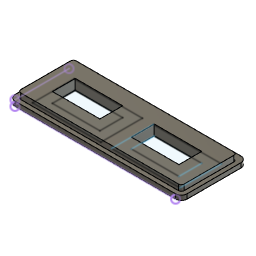
1593LBK_frontplate (Autodesk Fusion 360 design; units mm, degrees)
Autodesk Fusion 360 part; units mm, degrees
sketch "Skizze1" plane through (0, 0, 0) normal (0, 1, 0) x (1, 0, 0)
  arc A0 (0, 2) -> (2, 0) centre (2, 2) ccw
  arc A1 (2, 23) -> (0, 21) centre (2, 21) ccw
  line L0 (58.5, 23) -> (2, 23)
  line L1 (60.5, 2) -> (60.5, 21)
  arc A2 (58.5, 0) -> (60.5, 2) centre (58.5, 2) ccw
  line L2 (2, 0) -> (58.5, 0)
  line L3 (0, 21) -> (0, 2)
  arc A3 (60.5, 21) -> (58.5, 23) centre (58.5, 21) ccw
  point P0 (60.5, 0)
  point P1 (0, 23)
  dimension "d1" = 60.5
  dimension "d2" = 23
  dimension "d3" = 2
  dimension "d4" = 2
  dimension "d5" = 2
  dimension "d6" = 2
  constraint horizontal L2
  constraint vertical L1
  constraint horizontal L0
  constraint vertical L3
  constraint tangent L1 A3
  constraint tangent L0 A3
  constraint coincident P0 L2
  constraint coincident P0 L1
  constraint tangent A2 L2
  constraint tangent L1 A2
  constraint coincident origin L2
  constraint coincident origin L3
  constraint tangent A0 L2
  constraint tangent A0 L3
  constraint coincident P1 L0
  constraint coincident P1 L3
  constraint tangent A1 L0
  constraint tangent A1 L3
  measures "d1" distance of origin P0
  measures "d2" distance of origin P1
  measures "d3" radius of A3
  measures "d4" radius of A2
  measures "d5" radius of A0
  measures "d6" radius of A1
sketch "Skizze2" plane through (0, 0, 0) normal (0, 1, 0) x (1, 0, 0)
  line L0 (2.5, 1.5) -> (58, 1.5)
  line L1 (59, 2.5) -> (59, 20)
  line L2 (58, 21) -> (2.5, 21)
  line L3 (1.5, 20) -> (1.5, 2.5)
  line L4 (2, 0) -> (58.5, 0)
  line L5 (0, 21) -> (0, 2)
  arc A0 (2.5, 21) -> (1.5, 20) centre (2.5, 20) ccw
  arc A1 (1.5, 2.5) -> (2.5, 1.5) centre (2.5, 2.5) ccw
  arc A2 (59, 20) -> (58, 21) centre (58, 20) ccw
  arc A3 (58, 1.5) -> (59, 2.5) centre (58, 2.5) ccw
  point P0 (1.5, 1.5)
  point P1 (59, 1.5)
  point P2 (1.5, 21)
  dimension "d7" = 57.5
  dimension "d8" = 19.5
  dimension "d9" = 1.5
  dimension "d10" = 1.5
  dimension "d11" = 1
  constraint horizontal L0
  constraint vertical L1
  constraint horizontal L2
  constraint vertical L3
  constraint coincident P2 L2
  constraint coincident P2 L3
  constraint tangent L2 A0
  constraint tangent L3 A0
  constraint coincident P0 L0
  constraint coincident P0 L3
  constraint tangent L0 A1
  constraint tangent L3 A1
  constraint equal A0 A1
  constraint tangent L1 A2
  constraint tangent L2 A2
  constraint equal A0 A2
  constraint coincident P1 L0
  constraint coincident P1 L1
  constraint tangent L0 A3
  constraint tangent L1 A3
  constraint equal A0 A3
  measures "d7" distance of P0 P1
  measures "d8" distance of P0 P2
  measures "d9" distance of L0 L4
  measures "d10" distance of L3 L5
  measures "d11" radius of A0
sketch "Skizze5" plane through (0, 0, 0) normal (0, 1, 0) x (1, 0, 0)
  line L0 (4, 4.2) -> (28, 4.2)
  line L1 (28, 4.2) -> (28, 18.8)
  line L2 (28, 18.8) -> (4, 18.8)
  line L3 (4, 18.8) -> (4, 4.2)
  line L4 (7.65, 7.5) -> (24.35, 7.5)
  line L5 (24.35, 7.5) -> (24.35, 15.5)
  line L6 (24.35, 15.5) -> (7.65, 15.5)
  line L7 (7.65, 15.5) -> (7.65, 7.5)
  line L8 (0, 21) -> (0, 2)
  line L9 (35.45, 7.5) -> (52.15, 7.5)
  line L10 (52.15, 15.5) -> (35.45, 15.5)
  line L11 (35.45, 15.5) -> (35.45, 7.5)
  line L12 (55.8, 4.2) -> (55.8, 18.8)
  line L13 (55.8, 18.8) -> (31.8, 18.8)
  line L14 (31.8, 18.8) -> (31.8, 4.2)
  line L15 (31.8, 4.2) -> (55.8, 4.2)
  line L16 (2, 0) -> (58.5, 0)
  line L17 (52.15, 7.5) -> (52.15, 15.5)
  dimension "d52" = 24
  dimension "d53" = 14.6
  dimension "d54" = 16.7
  dimension "d55" = 8
  dimension "d56" = 3.3
  dimension "d57" = 3.65
  dimension "d58" = 4
  dimension "d59" = 24
  dimension "d60" = 14.6
  dimension "d61" = 16.7
  dimension "d62" = 8
  dimension "d63" = 3.3
  dimension "d65" = 4.2
  dimension "d66" = 4.2
  dimension "d81" = 3.65
  constraint horizontal L0
  constraint vertical L1
  constraint horizontal L2
  constraint vertical L3
  constraint horizontal L4
  constraint vertical L5
  constraint horizontal L6
  constraint vertical L7
  constraint horizontal L15
  constraint vertical L12
  constraint horizontal L13
  constraint vertical L14
  constraint horizontal L9
  constraint horizontal L10
  constraint vertical L11
  constraint perpendicular L10 L17
  measures "d52" distance of L0.start L0.end
  measures "d53" distance of L0.start L2.end
  measures "d54" distance of L4.start L4.end
  measures "d55" distance of L4.start L6.end
  measures "d56" distance of L2 L6
  measures "d57" distance of L3 L7
  measures "d58" distance of L3 L8
  measures "d59" distance of L14.end L12.start
  measures "d60" distance of L13.end L14.end
  measures "d61" distance of L9.start L9.end
  measures "d62" distance of L9.start L10.end
  measures "d63" distance of L10 L13
  measures "d65" distance of L0 L16
  measures "d66" distance of L15 L16
  measures "d81" distance of L12 L17
extrude "Extrusion8" add sketch "Skizze1" along normal blind 1.6
extrude "Extrusion9" add sketch "Skizze2" along normal blind 3.6
extrude "Extrusion10" cut sketch "Skizze5" along normal blind 20 contours L4 L5 L6 L7 | L9 L10 L11 L17
sketch "Skizze4" plane through (0, 0, 0) normal (0, 1, 0) x (1, 0, 0)
  circle A0 centre (44.5, 8) radius 1.5
  circle A1 centre (49.5, 8) radius 1.5
  circle A2 centre (54.5, 8) radius 1.5
  line L0 (2.5, 1.5) -> (58, 1.5)
  line L1 (24, 17.25) -> (24, 6.05)
  line L2 (36.5, 6.05) -> (36.5, 17.25)
  line L3 (2, 0) -> (58.5, 0)
  dimension "d16" = 3
  dimension "d17" = 3
  dimension "d18" = 3
  dimension "d19" = 5
  dimension "d20" = 5
  dimension "d25" = 8
  dimension "d26" = 8
  measures "d16" diameter of A0
  measures "d17" diameter of A1
  measures "d18" diameter of A2
  measures "d19" distance of A0.centre A1.centre
  measures "d20" distance of A1.centre A2.centre
  measures "d25" distance of A0.centre L2
  measures "d26" distance of A1.centre L3
extrude "Extrusion1" [suppressed]
extrude "Extrusion2" [suppressed]
extrude "Extrusion3" [suppressed]
equation "d16 = h1"
equation "d17 = h1"
equation "d18 = h1"
equation "h1 = 3 mm"
equation "h1_hoehe = 6.5 mm"
equation "d26 = h1_hoehe + ( h1 / 2 )"
